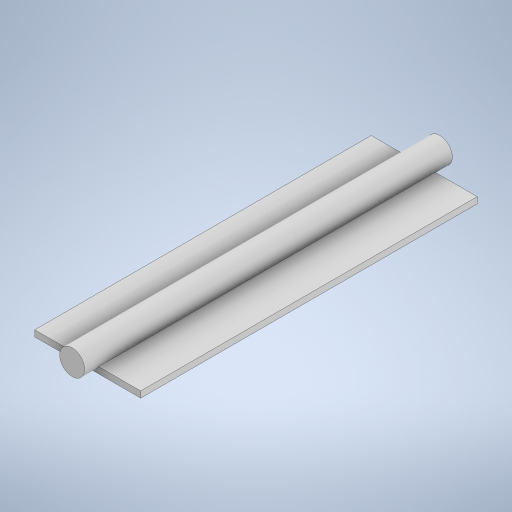
# Autodesk Inventor part: Air_Cotrol
Saved by Autodesk Inventor 2024.3 (Build 283343000, 343)
## iProperties
Created: 2025-03-09
Part Number: Air_Cotrol
Material: Generic
Document SubType Name: Modeling
Designer: ajclo
Density: 1 g/cm^3
Appearance: Default
Author: ajclo
Autodesk Inventor part; units mm, degrees
ref_plane "YZ Plane" through (0, 0, 0) normal (1, 0, 0) x (0, 1, 0)
ref_plane "XZ Plane" through (0, 0, 0) normal (0, 1, 0) x (-1, 0, 0)
ref_plane "XY Plane" through (0, 0, 0) normal (0, 0, 1) x (1, 0, 0)
sketch "Sketch1" plane through (0, 0, 0) normal (0, 1, 0) x (-1, 0, 0)
  line L0 (-17, 54) -> (17, 54)
  line L1 (17, 54) -> (17, -54)
  line L2 (17, -54) -> (-17, -54)
  line L3 (-17, -54) -> (-17, 54)
  line L4 (-17, 54) -> (17, -54) construction
  line L5 (17, 54) -> (-17, -54) construction
  point P0 (0, 0)
  dimension "d0" = 34
  dimension "d1" = 108
  constraints: 12 end point, 2 midpoint, 2 parallel, 1 horizontal, 1 perpendicular
  measures "d0" distance of L1.end L2.end
  measures "d1" distance of L0.end L1.end
extrude "Extrusion1" add sketch "Sketch1" along normal blind 2
sketch "Sketch2" plane through (0, 0, 0) normal (0, 0, 1) x (1, 0, 0)
  circle A0 centre (0, 4) radius 4
  point P0 (0, 0)
  dimension "d4" = 8
  constraints: 1 vertical alignment, 2 other
extrude "Extrusion2" add sketch "Sketch2" along normal mid plane 118
body "Solid1"
